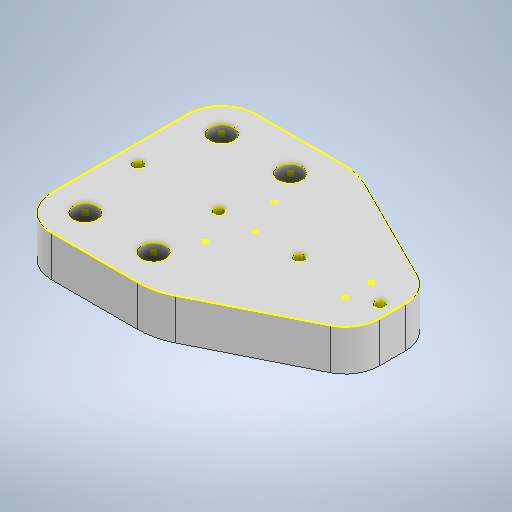
# Autodesk Inventor part: Linear_Mount
Saved by Autodesk Inventor 2025.1 (Build 291241020, 241B)
## iProperties
Created: 2024-11-27
Part Number: Linear_Mount
Material: Generic
Document SubType Name: Modeling
Designer: AtuStem
Density: 1 g/cm^3
Appearance: Default
Author: AtuStem
Autodesk Inventor part; units mm, degrees
ref_plane "YZ Plane" through (0, 0, 0) normal (1, 0, 0) x (0, 1, 0)
ref_plane "XZ Plane" through (0, 0, 0) normal (0, 1, 0) x (-1, 0, 0)
ref_plane "XY Plane" through (0, 0, 0) normal (0, 0, 1) x (1, 0, 0)
sketch "Sketch1" plane through (0, 0, 0) normal (0, 1, 0) x (-1, 0, 0)
  circle A0 centre (21.9, 0) radius 0.8
  circle A1 centre (6.9, 0) radius 0.8
  circle A2 centre (-8.1, 0) radius 0.8
  circle A3 centre (-23.1, 0) radius 0.8
  line L0 (25.4, -19.05) -> (-25.4, -19.05)
  line L1 (-25.4, 19.05) -> (-25.4, -19.05)
  line L2 (-25.4, 19.05) -> (25.4, 19.05)
  line L3 (25.4, -19.05) -> (25.4, 19.05)
  circle A4 centre (19.05, -12.7) radius 2.1844
  circle A5 centre (6.35, -12.7) radius 2.1844
  circle A6 centre (6.35, 12.7) radius 2.1844
  circle A7 centre (19.05, 12.7) radius 2.1844
  line L4 (25.4, 0) -> (-25.4, 0)
  line L5 (0, -19.05) -> (0, 19.05)
  circle A8 centre (0, 0) radius 1.235
  line L6 (-25.4, 0) -> (-25.4, 6.35)
  line L7 (-25.4, 6.35) -> (-25.4, -6.35)
  line L8 (0, 19.05) -> (-25.4, 6.35)
  line L9 (-25.4, -6.35) -> (0, -19.05)
  point P0 (21.9, 0)
  dimension "d3" = 1.6
  dimension "d4" = 1.6
  dimension "d5" = 1.6
  dimension "d6" = 1.6
  dimension "d7" = 6.35
  dimension "d8" = 12.7
  constraints: 20 end point, 9 centre point, 5 midpoint, 2 point on line
  measures "d3" diameter of A0
  measures "d4" diameter of A1
  measures "d5" diameter of A2
  measures "d6" diameter of A3
  measures "d7" distance of L4.end L6.end
  measures "d8" distance of L6.end L7.end
extrude "Extrusion1" add sketch "Sketch1" along normal blind 7.62 contours L4 L3 L0 L5 A8 A1 A0 | A0 L4 A1 A8 L5 L2 L3 | L9 L1 L4 A3 A2 A8 L5 | L5 A8 L4 A2 A3 L1 L8 | A8 L5 L4 | L4 L5 A8 | A8 L4 L5 | L5 L4 A8
fillet "Fillet1" radius 6.35 2 edges at (-25.4, 3.81, 19.05) (-25.4, 3.81, -19.05)
fillet "Fillet2" radius 6.35 2 edges at (25.4, 3.81, -6.35) (25.4, 3.81, 6.35)
fillet "Fillet3" radius 12.7 2 edges at (0, 3.81, -19.05) (0, 3.81, 19.05)
sketch "Sketch2" plane through (0, 7.62, 0) normal (0, 1, 0) x (1, 0, 0)
  arc A0 (-2.9981, -19.05) -> (2.6815, -17.7092) centre (-2.9981, -6.35) ccw projected
  line L0 (2.6815, -17.7092) -> (21.8898, -8.1051) projected
  arc A1 (21.8898, -8.1051) -> (25.4, -2.4255) centre (19.05, -2.4255) ccw projected
  line L1 (25.4, -2.4255) -> (25.4, 2.4255) projected
  arc A2 (25.4, 2.4255) -> (21.8898, 8.1051) centre (19.05, 2.4255) ccw projected
  line L2 (21.8898, 8.1051) -> (2.6815, 17.7092) projected
  arc A3 (2.6815, 17.7092) -> (-2.9981, 19.05) centre (-2.9981, 6.35) ccw projected
  line L3 (-2.9981, 19.05) -> (-19.05, 19.05) projected
  arc A4 (-19.05, 19.05) -> (-25.4, 12.7) centre (-19.05, 12.7) ccw projected
  line L4 (-25.4, 12.7) -> (-25.4, -12.7) projected
  arc A5 (-25.4, -12.7) -> (-19.05, -19.05) centre (-19.05, -12.7) ccw projected
  line L5 (-19.05, -19.05) -> (-2.9981, -19.05) projected
  circle A6 centre (-21.9, 0) radius 0.8 projected
  circle A7 centre (-6.9, 0) radius 0.8 projected
  circle A8 centre (-19.05, 12.7) radius 2.1844 projected
  circle A9 centre (-6.35, 12.7) radius 2.1844 projected
  circle A10 centre (23.1, 0) radius 0.8 projected
  circle A11 centre (8.1, 0) radius 0.8 projected
  circle A12 centre (-6.35, -12.7) radius 2.1844 projected
  circle A13 centre (-19.05, -12.7) radius 2.1844 projected
  circle A14 centre (-21.9, 0) radius 0.889
  circle A15 centre (-6.9, 0) radius 0.889
  circle A16 centre (8.1, 0) radius 0.889
  circle A17 centre (23.1, 0) radius 0.889
  point P0 (0, 0)
  dimension "d14" = 1.778
  dimension "d15" = 1.778
  dimension "d16" = 1.778
  dimension "d17" = 1.778
  constraints: 4 centre point, 4 coincident
  measures "d14" diameter of A14
  measures "d15" diameter of A15
  measures "d16" diameter of A16
  measures "d17" diameter of A17
extrude "Extrusion2" cut sketch "Sketch2" along normal through all both and the other way through all contours A14 | A15 | A16 | A17
sketch "Sketch3" plane through (0, 7.62, 0) normal (0, 1, 0) x (1, 0, 0)
  circle A0 centre (-6.9, 0) radius 0.889 projected
  circle A1 centre (8.1, 0) radius 0.889 projected
  circle A2 centre (-21.9, 0) radius 0.889 projected
  circle A3 centre (23.1, 0) radius 0.889 projected
  arc A4 (-2.9981, -19.05) -> (2.6815, -17.7092) centre (-2.9981, -6.35) ccw projected
  line L0 (2.6815, -17.7092) -> (21.8898, -8.1051) projected
  arc A5 (21.8898, -8.1051) -> (25.4, -2.4255) centre (19.05, -2.4255) ccw projected
  line L1 (25.4, -2.4255) -> (25.4, 2.4255) projected
  arc A6 (25.4, 2.4255) -> (21.8898, 8.1051) centre (19.05, 2.4255) ccw projected
  line L2 (21.8898, 8.1051) -> (2.6815, 17.7092) projected
  arc A7 (2.6815, 17.7092) -> (-2.9981, 19.05) centre (-2.9981, 6.35) ccw projected
  line L3 (-2.9981, 19.05) -> (-19.05, 19.05) projected
  arc A8 (-19.05, 19.05) -> (-25.4, 12.7) centre (-19.05, 12.7) ccw projected
  line L4 (-25.4, 12.7) -> (-25.4, -12.7) projected
  arc A9 (-25.4, -12.7) -> (-19.05, -19.05) centre (-19.05, -12.7) ccw projected
  line L5 (-19.05, -19.05) -> (-2.9981, -19.05) projected
  circle A10 centre (-19.05, 12.7) radius 2.1844 projected
  circle A11 centre (-6.35, 12.7) radius 2.1844 projected
  circle A12 centre (-6.35, -12.7) radius 2.1844 projected
  circle A13 centre (-19.05, -12.7) radius 2.1844 projected
  point P0 (0, 0)
body "Solid1"
